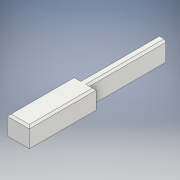
# Autodesk Inventor part: key_3
Saved by Autodesk Inventor 2017 (Build 210142000, 142)
## iProperties
Created: 2018-03-15
Part Number: key_3
Material: Generic
Document SubType Name: Modeling
Designer: Luiz Gustavo
Density: 1 g/cm^3
Appearance: White
Author: Luiz Gustavo
Autodesk Inventor part; units mm, degrees
ref_plane "YZ Plane" through (0, 0, 0) normal (1, 0, 0) x (0, 1, 0)
ref_plane "XZ Plane" through (0, 0, 0) normal (0, 1, 0) x (-1, 0, 0)
ref_plane "XY Plane" through (0, 0, 0) normal (0, 0, 1) x (1, 0, 0)
sketch "Sketch1" plane through (0, 0, 0) normal (0, 0, 1) x (1, 0, 0)
  line L0 (-11.5, -75) -> (11.5, -75)
  line L1 (11.5, -75) -> (11.5, 75)
  line L2 (11.5, 75) -> (-11.5, 75)
  line L3 (-11.5, 75) -> (-11.5, -75)
  line L4 (-11.5, -75) -> (11.5, 75) construction
  line L5 (11.5, -75) -> (-11.5, 75) construction
  line L6 (-4.5, 75) -> (4.5, 75)
  line L7 (4.5, 75) -> (4.5, -5)
  line L8 (4.5, -5) -> (-4.5, -5) construction
  line L9 (-4.5, -5) -> (-4.5, 75)
  line L10 (0, -75) -> (0, 75) construction
  line L11 (-4.5, -5) -> (-11.5, -5)
  line L12 (4.5, -5) -> (11.5, -5)
  point P0 (0, 0)
  dimension "d0" = 150
  dimension "d1" = 80
  dimension "d2" = 7
  dimension "d3" = 23
  constraints: 26 end point, 4 midpoint, 4 parallel, 3 perpendicular, 3 point on line, 2 horizontal, 1 collinear, 1 other
  measures "d0" distance of L0.end L1.end
  measures "d1" distance between parallel lines of L8 L2
  measures "d2" distance between parallel lines of L3 L9
  measures "d3" distance between parallel lines of L3 L1
extrude "Extrusion1" add sketch "Sketch1" against normal blind 20 contours L3 L11 L9 L2 L7 L12 L1 L0
chamfer "Chamfer1" distance 2 angle 45 7 edges at (0, -75, 0) (-11.5, -40, 0) (11.5, -40, 0) (8, -5, 0) (-8, -5, 0) (-4.5, 35, 0) (4.5, 35, 0)
equation "\"d0\" = key_length"
equation "\"d1\" = blackkey_length"
equation "\"d2\" = blackkey_halfwidth"
equation "\"d3\" = key_width"
equation "\"d4\" = key_height"
equation "\"key_length\" = 150"
equation "\"blackkey_length\" = 80"
equation "\"blackkey_halfwidth\" = 7"
equation "\"key_width\" = 23"
equation "\"key_height\" = 20"
body "Solid1"
